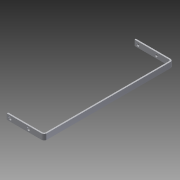
# Autodesk Inventor part: tie-together tier 2 wide
Saved by Autodesk Inventor 2013 (Build 170138000, 138)
## iProperties
Created: 2013-01-24
Part Number: tie-together tier 2 wide
Material: Aluminum 6061
Document SubType Name: Sheet Metal
Designer: Arpan
Density: 2.71 g/cm^3
Sheet Metal Rule: Default
Mass: 28.8234 g
Surface Area: 87.8738 cm^2
Volume: 10.6359 cm^3
Author: Arpan
Autodesk Inventor part; units mm, degrees
ref_plane "YZ Plane" through (0, 0, 0) normal (1, 0, 0) x (0, 1, 0)
ref_plane "XZ Plane" through (0, 0, 0) normal (0, 1, 0) x (-1, 0, 0)
ref_plane "XY Plane" through (0, 0, 0) normal (0, 0, 1) x (1, 0, 0)
sketch "Sketch1" plane through (0, 0, 0) normal (0, 0, 1) x (1, 0, 0)
  line L0 (0, 0) -> (-79.2226, 0)
  line L1 (-79.2226, 0) -> (-79.2226, 12.7)
  line L2 (-79.2226, 12.7) -> (0, 12.7)
  line L3 (0, 12.7) -> (0, 0)
  line L4 (0, 12.7) -> (-29.718, 12.7)
  line L5 (-79.2226, 12.7) -> (-71.7296, 12.7)
  dimension "d1" = 79.2226
  dimension "d2" = 12.7
  dimension "d5" = 7.493
  constraints: 12 end point, 2 perpendicular, 2 point on line, 1 horizontal, 1 parallel
  measures "d1" distance of L0.start L0.end
  measures "d2" distance of L0.end L1.end
  measures "d5" distance of L1.end L5.end
extrude "Plate5" add sketch "Sketch1" along normal blind 3.175
sketch "Sketch6" plane through (3.175, 0, -3.175) normal (1, 0, 0) x (0, 1, 0)
  line L0 (12.7, 0) -> (0, 0)
  line L1 (0, 0) -> (0, -283.0322)
  line L2 (0, -283.0322) -> (12.7, -283.0322)
  line L3 (12.7, -283.0322) -> (12.7, 0)
  constraints: 6 end point, 1 horizontal, 1 perpendicular, 1 vertical
edge flange "Flange4" height 289.3822 angle 90 thickness 3.175 bend radius 3.175 thickness toward (1, 0, 0) relief straight relief width 3.175 relief depth 1.5875 edges at (0, 6.35, 0) wall of the first edge with corners at (3.175, 12.7, -3.175) (3.175, 0, -3.175) (3.175, 0, -286.2072) (3.175, 12.7, -286.2072)
bend "Bend4"
corner "Corner4"
sketch "Sketch7" plane through (0, 0, -289.3822) normal (0, 0, -1) x (-1, 0, 0)
  line L0 (0, 12.7) -> (0, 0)
  line L1 (0, 0) -> (79.2226, 0)
  line L2 (79.2226, 0) -> (79.2226, 12.7)
  line L3 (79.2226, 12.7) -> (0, 12.7)
  constraints: 6 end point, 1 horizontal, 1 perpendicular, 1 vertical
edge flange "Flange5" height 85.5726 angle 90 thickness 3.175 bend radius 3.175 thickness toward (0, 0, -1) relief straight relief width 3.175 relief depth 1.5875 edges at (3.175, 6.35, -286.2072) wall of the first edge with corners at (0, 12.7, -289.3822) (0, 0, -289.3822) (-79.2226, 0, -289.3822) (-79.2226, 12.7, -289.3822)
bend "Bend5"
corner "Corner5"
sketch "Sketch8" plane through (0, 0, 3.175) normal (0, 0, 1) x (1, 0, 0)
  circle A0 centre (-71.725, 5.9188) radius 3.3 projected
  circle A1 centre (-29.725, 5.9188) radius 3.3 projected
extrude "Extrusion2" cut sketch "Sketch8" against normal blind 2539974.6
equation "\"d43\" = BendReliefWidth"
equation "\"d44\" = BendReliefDepth"
equation "\"d45\" = MinimumRemnant"
equation "\"d46\" = BendRadius"
equation "\"d49\" = BendRadius"
equation "\"d50\" = CornerReliefSize"
equation "\"d51\" = GapSize"
equation "\"d52\" = JacobiRadiusSize"
equation "\"d53\" = BendReliefWidth"
equation "\"d54\" = BendReliefDepth"
equation "\"d55\" = MinimumRemnant"
equation "\"d56\" = BendRadius"
equation "\"d59\" = BendRadius"
equation "\"d60\" = CornerReliefSize"
equation "\"d61\" = GapSize"
equation "\"d62\" = JacobiRadiusSize"
equation "\"BendRadius\" = Thickness"
equation "\"BendReliefWidth\" = Thickness"
equation "\"BendReliefDepth\" = 0.5 * Thickness"
equation "\"CornerReliefSize\" = 4 * Thickness"
equation "\"MinimumRemnant\" = 2 * Thickness"
equation "\"TransitionRadius\" = BendRadius"
equation "\"JacobiRadiusSize\" = BendRadius"
equation "\"GapSize\" = Thickness"
equation "\"d8\" = BendRadius"
equation "\"d42\" = BendRadius"
equation "\"Thickness\" = 3.175"
body "Solid2"
